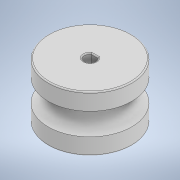
# Autodesk Inventor part: DriveWheelHalf
Saved by Autodesk Inventor 2021 (Build 250183000, 183)
## iProperties
Created: 2021-07-08
Part Number: DriveWheelHalf
Material: Generic
Document SubType Name: Modeling
Designer: zmac845
Density: 1 g/cm^3
Appearance: Default
Author: zmac845
Autodesk Inventor part; units mm, degrees
ref_plane "YZ Plane" through (0, 0, 0) normal (1, 0, 0) x (0, 1, 0)
ref_plane "XZ Plane" through (0, 0, 0) normal (0, 1, 0) x (-1, 0, 0)
ref_plane "XY Plane" through (0, 0, 0) normal (0, 0, 1) x (1, 0, 0)
sketch "Sketch1" plane through (0, 0, 0) normal (0, 0, 1) x (1, 0, 0)
  line L0 (0, 0) -> (18, 0)
  line L1 (18, 0) -> (18, 12)
  line L2 (18, 12) -> (0, 12)
  line L3 (0, 12) -> (0, 0)
  line L4 (0, 0) -> (11, 0)
  line L5 (11, 12) -> (0, 12)
  line L6 (0, 12) -> (0, 0)
  line L7 (18, 12) -> (19.5, 12)
  arc A0 (14.5, 12) -> (22.6054, 8.0813) centre (19.5, 12) ccw
  point P0 (18, 7.2303)
  dimension "d0" = 18
  dimension "d1" = 12
  dimension "d3" = 1.5
  dimension "d4" = 5
  constraints: 16 end point, 3 parallel, 2 horizontal, 2 perpendicular, 2 point on circle, 2 point on line, 1 centre point, 1 coincident
  measures "d0" distance of L2.end L1.end
  measures "d1" distance of L1.end L0.end
  measures "d3" distance of L1.end L7.end
  measures "d4" radius of A0
revolve "Revolution1" add sketch "Sketch1" angle 360 about axis through (0, 12, 0) along (0, -1, 0) contours L3 L2 A0 L1 L0
mirror "Mirror1" about plane through (14.5, 12, 0) normal (0, 1, 0) of "Revolution1"
fillet "Fillet1" radius 0.5 2 edges at (-18, 0, 0) (-18, 24, 0)
sketch "Sketch2" plane through (0, 24, 0) normal (0, 1, 0) x (1, 0, 0)
  arc A0 (-1.5, 2) -> (1.5, 2) centre (0, 0) ccw
  line L0 (-1.5, 2) -> (1.5, 2)
  dimension "d7" = 5
  dimension "d8" = 2
  constraints: 2 end point, 2 point on circle, 1 centre point, 1 coincident, 1 horizontal
  measures "d7" diameter of A0
  measures "d8" distance from line of point (0, 0) L0
extrude "Extrusion1" cut sketch "Sketch2" against normal blind 12.25
sketch "Sketch3" plane through (0, 0, 0) normal (0, -1, 0) x (1, 0, 0)
  circle A0 centre (0, 0) radius 4
  dimension "d11" = 8
  constraints: 1 centre point, 1 coincident
  measures "d11" diameter of A0
extrude "Extrusion2" cut sketch "Sketch3" against normal blind 11.75
sketch "Sketch4" plane through (0, 0, 0) normal (0, -1, 0) x (1, 0, 0)
  line L0 (6.5352, 3.6912) -> (6.4642, -3.8141)
  line L1 (6.4642, -3.8141) -> (-0.0709, -7.5052)
  line L2 (-0.0709, -7.5052) -> (-6.5352, -3.6912)
  line L3 (-6.5352, -3.6912) -> (-6.4642, 3.8141)
  line L4 (-6.4642, 3.8141) -> (0.0709, 7.5052)
  line L5 (0.0709, 7.5052) -> (6.5352, 3.6912)
  point P0 (0, 0)
  point P1 (0, 0)
  dimension "d14" = 13
  constraints: 12 end point, 1 coincident, 13 other
  measures "d14" distance between parallel lines of L3 L0
extrude "Extrusion3" cut sketch "Sketch4" against normal blind 7
fillet "Fillet2" radius 0.5 11 edges at (-3.3031, 0, -5.5982) (3.1966, 0, -5.6596) (6.4997, 0, -0.0614) (3.3031, 0, 5.5982) (-3.1966, 0, 5.6596) (-6.4997, 0, 0.0614) (-4, 7, 0) (0, 11.75, -2) (0, 11.75, 2.5) (0, 24, 2.5) (0, 24, -2)
body "Solid1"
